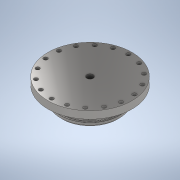
# Autodesk Inventor part: ODSY-0003-201
Saved by Autodesk Inventor 2021 (Build 250183000, 183)
## iProperties
Company: ERPL
Created: 2021-09-22
Part Number: ODSY-0003-201
Material: Stainless Steel
Document SubType Name: Modeling
Designer: ALEX CLAY
Density: 8 g/cm^3
Appearance: Semi-Polished
Mass: 2164.69 g
Surface Area: 618.631 cm^2
Volume: 270.587 cm^3
Project: ODYSSEY
Description: INJECTOR MANIFOLD
Author: ALEX CLAY
Revision Number: 00
Autodesk Inventor part; units mm, degrees
ref_plane "YZ Plane" through (0, 0, 0) normal (1, 0, 0) x (0, 1, 0)
ref_plane "XZ Plane" through (0, 0, 0) normal (0, 1, 0) x (-1, 0, 0)
ref_plane "XY Plane" through (0, 0, 0) normal (0, 0, 1) x (1, 0, 0)
sketch "Sketch1" plane through (0, 0, 0) normal (0, 1, 0) x (-1, 0, 0)
  circle A0 centre (0, 0) radius 73.025
  dimension "d0" = 146.05
  constraints: 1 centre point, 1 coincident
  measures "d0" diameter of A0
extrude "Extrusion1" add sketch "Sketch1" along normal blind 12.7
sketch "Sketch2" plane through (0, 12.7, 0) normal (0, 1, 0) x (1, 0, 0)
  point P0 (0, 0)
  point P1 (0, 66.675)
  dimension "d10" = 66.675
  constraints: 1 vertical alignment
  measures "d10" distance of point (0, 0) point (0, 66.675)
hole "Hole1" at (0, 12.7, -66.675) direction (0, -1, 0) diameter 6.7564 end through all clearance for "Flat Head Machine Screw (82)" size "1/4" standard "Ansi Unified Screw Threads"
pattern_circular "Circular Pattern1" count 18 over 360 about axis through (0, 0, 0) along (0, 1, 0) of "Hole1"
sketch "Sketch3" plane through (0, 0, 0) normal (0, -1, 0) x (1, 0, 0)
  circle A0 centre (0, 0) radius 50.8
  circle A1 centre (0, 0) radius 41.275
  dimension "d14" = 101.6
  dimension "d15" = 82.55
  constraints: 2 centre point, 2 coincident
  measures "d14" diameter of A0
  measures "d15" diameter of A1
extrude "Extrusion2" add sketch "Sketch3" along normal blind 27.94
sketch "Sketch5" plane through (0, 12.7, 0) normal (0, 1, 0) x (1, 0, 0)
  point P0 (0, 0)
hole "Hole2" at (0, 12.7, 0) direction (0, -1, 0) diameter 10.7188 end through all taper from width 11.3583 to width 10.7323 over 10.0203 thread size "1/4" designation "1/4 - 18 NPT" standard "NPT"
sketch "Sketch6" plane through (0, 0, 0) normal (0, -1, 0) x (1, 0, 0)
  line L0 (0, 0) -> (0, -28.575) construction
  dimension "d42" = 28.575
  constraints: 2 end point, 1 vertical alignment
  measures "d42" distance of L0.start L0.end
hole "Hole3" at (0, 0, -28.575) direction (0, 1, 0) diameter 4.9784 depth 10.16 thread size "1/4-20 UNC" class "2B" standard "ANSI Unified Screw Threads"
pattern_circular "Circular Pattern2" count 6 over 360 about axis through (0, 0, 0) along (0, -1, 0) of "Hole3"
chamfer "Chamfer3" distance 3.175 angle 45 1 edges at (-50.8, -27.94, 0)
sketch "Sketch9" plane through (0, 0, 0) normal (0, 0, 1) x (1, 0, 0)
  line L0 (47.625, -27.94) -> (-47.625, -27.94) projected
  line L1 (-50.8, -20.7899) -> (-48.4886, -20.7899)
  line L2 (-47.9806, -20.2819) -> (-47.9806, -16.5481)
  line L3 (-48.4886, -16.0401) -> (-50.8, -16.0401)
  line L4 (-50.8, -16.0401) -> (-50.8, -20.7899)
  line L5 (-50.8, -14.4399) -> (-48.4886, -14.4399)
  line L6 (-47.9806, -13.9319) -> (-47.9806, -10.1981)
  line L7 (-48.4886, -9.6901) -> (-50.8, -9.6901)
  line L8 (-50.8, -9.6901) -> (-50.8, -14.4399)
  line L9 (0, -33.528) -> (0, 5.588) projected
  line L10 (-47.9806, -12.065) -> (-56.5456, -12.065) construction
  line L11 (-47.9806, -18.415) -> (-55.9743, -18.415) construction
  arc A0 (-47.9806, -10.1981) -> (-48.4886, -9.6901) centre (-48.4886, -10.1981) ccw
  arc A1 (-48.4886, -14.4399) -> (-47.9806, -13.9319) centre (-48.4886, -13.9319) ccw
  arc A2 (-47.9806, -16.5481) -> (-48.4886, -16.0401) centre (-48.4886, -16.5481) ccw
  arc A3 (-48.4886, -20.7899) -> (-47.9806, -20.2819) centre (-48.4886, -20.2819) ccw
  point P0 (0, 0)
  point P1 (-47.9806, -16.0401)
  point P2 (-47.9806, -20.7899)
  point P3 (-47.9806, -9.6901)
  point P4 (-47.9806, -14.4399)
  dimension "d64" = 4.7498
  dimension "d65" = 4.7498
  dimension "d72" = 9.525
  dimension "d73" = 6.35
  dimension "d75" = 50.8
  dimension "d76" = 0.508
  dimension "d77" = 0.508
  dimension "d78" = 0.508
  dimension "d80" = 2.8194
  constraints: 20 end point, 10 point on line, 8 point on circle, 8 tangent, 4 centre point, 4 horizontal, 4 parallel, 2 midpoint, 2 perpendicular, 1 equal radius
  measures "d64" distance of point (-47.981, -14.44) point (-47.981, -9.69)
  measures "d65" distance of point (-47.981, -20.79) point (-47.981, -16.04)
  measures "d72" distance between parallel lines of L11 L0
  measures "d73" distance between parallel lines of L11 L10
  measures "d75" distance between parallel lines of L9 L4
  measures "d76" radius of A0
  measures "d77" radius of A1
  measures "d78" radius of A2
  measures "d80" distance between parallel lines of L2 L4
revolve "Revolution3" cut sketch "Sketch9" angle 360 about axis through (0, -10, 0) along (0, 1, 0)
fillet "Fillet1" radius 3.175 2 edges at (-50.8, 0, 0) (-41.275, 0, 0)
ref_plane "Work Plane1" through (0, -12.065, 0) normal (0, 1, 0) x (1, 0, 0)
ref_plane "Work Plane2" through (0, -18.415, 0) normal (0, 1, 0) x (1, 0, 0)
fillet "Fillet2" radius 0.127 4 edges at (-50.8, -9.6901, 0) (-50.8, -14.4399, 0) (-50.8, -16.0401, 0) (-50.8, -20.7899, 0)
body "Solid1"
